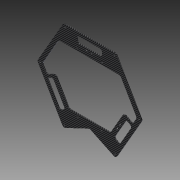
# Autodesk Inventor part: Bottom Plate
Saved by Autodesk Inventor 2015 (Build 190159000, 159)
## iProperties
Created: 2016-10-01
Part Number: Bottom Plate
Material: Generic
Document SubType Name: Modeling
Designer: James Yelland
Density: 1 g/cm^3
Appearance: Default
Mass: 19.8177 g
Surface Area: 231.547 cm^2
Volume: 19.8177 cm^3
Author: James Yelland
Autodesk Inventor part; units mm, degrees
ref_plane "YZ Plane" through (0, 0, 0) normal (1, 0, 0) x (0, 1, 0)
ref_plane "XZ Plane" through (0, 0, 0) normal (0, 1, 0) x (-1, 0, 0)
ref_plane "XY Plane" through (0, 0, 0) normal (0, 0, 1) x (1, 0, 0)
sketch "Sketch1" plane through (0, 0, 0) normal (0, 1, 0) x (-1, 0, 0)
  line L0 (72.6878, -41.9663) -> (62.1878, -60.1529)
  line L1 (72.6878, -41.9663) -> (83.1878, -23.7798)
  line L2 (81.7237, -18.3157) -> (77.3936, -15.8157)
  line L3 (71.9295, -17.2797) -> (50.9295, -53.6529)
  line L4 (52.3936, -59.117) -> (56.7237, -61.617)
  arc A0 (56.7237, -61.617) -> (62.1878, -60.1529) centre (58.7237, -58.1529) ccw
  arc A1 (50.9295, -53.6529) -> (52.3936, -59.117) centre (54.3936, -55.6529) ccw
  arc A2 (77.3936, -15.8157) -> (71.9295, -17.2797) centre (75.3936, -19.2798) ccw
  arc A3 (83.1878, -23.7798) -> (81.7237, -18.3157) centre (79.7237, -21.7798) ccw
  line L5 (55.5994, -35.5644) -> (57.3314, -36.5644)
  line L6 (57.3314, -36.5644) -> (54.8314, -40.8945)
  line L7 (53.0994, -39.8945) -> (55.5994, -35.5644)
  line L8 (54.8314, -40.8945) -> (53.0994, -39.8945)
  line L9 (61.0994, -26.0381) -> (58.5994, -30.3683)
  line L10 (60.3314, -31.3683) -> (62.8314, -27.0381)
  line L11 (58.5994, -30.3683) -> (60.3314, -31.3683)
  line L12 (62.8314, -27.0381) -> (61.0994, -26.0381)
  line L13 (0, 83.9327) -> (21, 83.9327)
  line L14 (0, 83.9327) -> (-21, 83.9327)
  line L15 (-25, 79.9327) -> (-25, 74.9327)
  line L16 (-21, 70.9327) -> (20.9998, 70.9327)
  line L17 (25, 74.9327) -> (25, 79.9327)
  arc A4 (25, 79.9327) -> (21, 83.9327) centre (21, 79.9327) ccw
  arc A5 (20.9998, 70.9327) -> (25, 74.9327) centre (21, 74.9327) ccw
  arc A6 (-25, 74.9327) -> (-21, 70.9327) centre (-21, 74.9327) ccw
  arc A7 (-21, 83.9327) -> (-25, 79.9327) centre (-21, 79.9327) ccw
  line L18 (3, 65.9327) -> (3, 67.9327)
  line L19 (8, 65.9327) -> (3, 65.9327)
  line L20 (8, 67.9327) -> (8, 65.9327)
  line L21 (3, 67.9327) -> (8, 67.9327)
  line L22 (-8, 67.9327) -> (-8, 65.9327)
  line L23 (-8, 65.9327) -> (-3, 65.9327)
  line L24 (-3, 65.9327) -> (-3, 67.9327)
  line L25 (-3, 67.9327) -> (-8, 67.9327)
  line L26 (-72.6878, -41.9663) -> (-83.1878, -23.7798)
  line L27 (-72.6878, -41.9663) -> (-62.1878, -60.1529)
  line L28 (-56.7237, -61.617) -> (-52.3936, -59.117)
  line L29 (-50.9295, -53.6529) -> (-71.9294, -17.28)
  line L30 (-77.3936, -15.8157) -> (-81.7237, -18.3157)
  arc A8 (-81.7237, -18.3157) -> (-83.1878, -23.7798) centre (-79.7237, -21.7798) ccw
  arc A9 (-71.9294, -17.28) -> (-77.3936, -15.8157) centre (-75.3936, -19.2798) ccw
  arc A10 (-52.3936, -59.117) -> (-50.9295, -53.6529) centre (-54.3936, -55.6529) ccw
  arc A11 (-62.1878, -60.1529) -> (-56.7237, -61.617) centre (-58.7237, -58.1529) ccw
  line L31 (-58.5994, -30.3683) -> (-60.3314, -31.3683)
  line L32 (-61.0994, -26.0381) -> (-58.5994, -30.3683)
  line L33 (-62.8314, -27.0381) -> (-61.0994, -26.0381)
  line L34 (-60.3314, -31.3683) -> (-62.8314, -27.0381)
  line L35 (-54.8314, -40.8945) -> (-53.0994, -39.8945)
  line L36 (-53.0994, -39.8945) -> (-55.5994, -35.5644)
  line L37 (-55.5994, -35.5644) -> (-57.3314, -36.5644)
  line L38 (-57.3314, -36.5644) -> (-54.8314, -40.8945)
  line L39 (103.5566, -2.5) -> (54.8095, -86.9325)
  line L40 (-54.8095, -86.9325) -> (-103.5566, -2.5)
  line L41 (-103.5566, 2.5) -> (-53.9434, 88.4327)
  line L42 (-49.6132, 90.9327) -> (49.6132, 90.9327)
  line L43 (53.9434, 88.4327) -> (103.5566, 2.5)
  line L44 (2.1497, -66.9563) -> (48.3297, -88.9468)
  line L45 (-2.1497, -66.9563) -> (-48.3297, -88.9468)
  arc A12 (48.3297, -88.9468) -> (54.8095, -86.9325) centre (50.4794, -84.4325) ccw
  arc A13 (2.1497, -66.9563) -> (-2.1497, -66.9563) centre (0, -71.4706) ccw
  arc A14 (-54.8095, -86.9325) -> (-48.3297, -88.9468) centre (-50.4794, -84.4325) ccw
  arc A15 (-103.5566, 2.5) -> (-103.5566, -2.5) centre (-99.2265, 0) ccw
  arc A16 (-49.6132, 90.9327) -> (-53.9434, 88.4327) centre (-49.6132, 85.9327) ccw
  arc A17 (53.9434, 88.4327) -> (49.6132, 90.9327) centre (49.6132, 85.9327) ccw
  arc A18 (103.5566, -2.5) -> (103.5566, 2.5) centre (99.2265, 0) ccw
  circle A19 centre (49.6132, 85.9327) radius 1.6
  circle A20 centre (-49.6132, 85.9327) radius 1.6
  circle A21 centre (-99.2265, 0) radius 1.6
  circle A22 centre (99.2265, 0) radius 1.6
  line L46 (-88.75, -10.8253) -> (-93.5566, -2.5)
  arc A23 (-88.75, -10.8253) -> (-81.9199, -12.6554) centre (-84.4199, -8.3253) ccw
  arc A24 (-93.5566, 2.5) -> (-93.5566, -2.5) centre (-89.2265, 0) ccw
  line L47 (88.75, -10.8253) -> (93.5566, -2.5)
  arc A25 (81.9199, -12.6554) -> (88.75, -10.8253) centre (84.4199, -8.3253) ccw
  arc A26 (93.5566, -2.5) -> (93.5566, 2.5) centre (89.2265, 0) ccw
  line L48 (81.9199, -12.6554) -> (73.2596, -7.6554)
  line L49 (-81.9199, -12.6554) -> (-73.2596, -7.6554)
  arc A27 (73.2596, -7.6554) -> (66.4295, -9.4856) centre (70.7596, -11.9856) ccw
  arc A28 (-66.4295, -9.4856) -> (-73.2596, -7.6554) centre (-70.7596, -11.9856) ccw
  line L50 (0, -52.117) -> (-38.9295, -52.117)
  line L51 (0, -52.117) -> (38.9295, -52.117)
  line L52 (66.4295, -9.4856) -> (43.2596, -49.617)
  line L53 (-43.2596, -49.617) -> (-66.4295, -9.4856)
  arc A29 (38.9295, -52.117) -> (43.2596, -49.617) centre (38.9295, -47.117) ccw
  arc A30 (-43.2596, -49.617) -> (-38.9295, -52.117) centre (-38.9295, -47.117) ccw
  circle A31 centre (50.4794, -84.4325) radius 1.6
  circle A32 centre (-50.4794, -84.4325) radius 1.6
  line L54 (0, 57.2724) -> (-59.047, 57.2724)
  line L55 (0, 57.2724) -> (59.047, 57.2724)
  line L56 (93.5566, 2.5) -> (63.3771, 54.7724)
  line L57 (-63.3771, 54.7724) -> (-93.5566, 2.5)
  arc A33 (-59.047, 57.2724) -> (-63.3771, 54.7724) centre (-59.047, 52.2724) ccw
  arc A34 (63.3771, 54.7724) -> (59.047, 57.2724) centre (59.047, 52.2724) ccw
  circle A35 centre (-25, 62.282) radius 1.6
  circle A36 centre (25, 62.282) radius 1.6
  circle A37 centre (24, -57.282) radius 1.6
  circle A38 centre (-24, -57.282) radius 1.6
  point P0 (60.1878, -63.617)
  point P1 (85.1878, -20.3157)
  point P2 (73.9295, -13.8157)
  point P3 (48.9295, -57.117)
  point P4 (25, 83.9327)
  point P5 (-25, 83.9327)
  point P6 (-25, 70.9327)
  point P7 (25, 70.9327)
  point P8 (-85.1878, -20.3157)
  point P9 (-60.1878, -63.617)
  point P10 (-48.9295, -57.117)
  point P11 (-73.9295, -13.8157)
  point P12 (105, 0)
  point P13 (52.5, -90.9327)
  point P14 (-105, 0)
  point P15 (-52.5, 90.9327)
  point P16 (52.5, 90.9327)
  point P17 (-86.25, -15.1554)
  point P18 (68.9295, -5.1554)
  point P19 (61.9338, 57.2724)
  dimension "d11" = 360
  dimension "d30" = 360
  dimension "d72" = 5
  dimension "d75" = 3.2
  dimension "d76" = 3.2
  dimension "d78" = 5
  dimension "d83" = 3.2
  dimension "d84" = 3.2
  dimension "d85" = 3.2
  dimension "d86" = 3.2
  constraints: 116 end point, 58 point on circle, 39 centre point, 38 point on line, 9 tangent, 6 coincident, 2 equal radius, 1 horizontal
  measures "d72" radius of A29
  measures "d75" diameter of A31
  measures "d76" diameter of A32
  measures "d78" radius of A33
  measures "d83" diameter of A35
  measures "d84" diameter of A36
  measures "d85" diameter of A37
  measures "d86" diameter of A38
extrude "Extrusion1" add sketch "Sketch1" along normal blind 2
body "Solid1"
